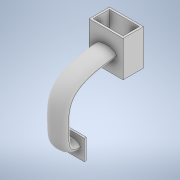
# Autodesk Inventor part: Verbindung_Motor_Servo
Saved by Autodesk Inventor 2021 (Build 250183000, 183)
## iProperties
Created: 2021-01-04
Part Number: Verbindung_Motor_Servo
Material: Generisch
Document SubType Name: Modeling
Designer: Ctroi
Density: 1 g/cm^3
Appearance: Vorgabe
Author: Ctroi
Autodesk Inventor part; units mm, degrees
ref_plane "YZ Plane" through (0, 0, 0) normal (1, 0, 0) x (0, 1, 0)
ref_plane "XZ Plane" through (0, 0, 0) normal (0, 1, 0) x (-1, 0, 0)
ref_plane "XY Plane" through (0, 0, 0) normal (0, 0, 1) x (1, 0, 0)
sketch "Skizze1" plane through (0, 0, 0) normal (0, 1, 0) x (-1, 0, 0)
  line L0 (25, -15) -> (-25, -15)
  line L1 (-25, -15) -> (-25, 15)
  line L2 (-25, 15) -> (25, 15)
  line L3 (25, 15) -> (25, -15)
  line L4 (35, 0) -> (-35, 0) projected
  line L5 (0, -21) -> (0, 21) projected
  point P0 (0, 0)
  dimension "d0" = 50
  dimension "d1" = 30
  constraints: 8 end point, 2 parallel, 1 horizontal, 1 perpendicular, 2 other
  measures "d0" distance of L1.end L2.end
  measures "d1" distance of L0.end L1.end
extrude "Extrusion1" add sketch "Skizze1" along normal blind 3
sketch "Skizze2" plane through (0, 3, 0) normal (0, 1, 0) x (1, 0, 0)
  line L0 (25, -15) -> (25, 15) projected
  line L1 (-25, 15) -> (-25, -15) projected
  line L2 (25, 15) -> (-25, 15)
  line L3 (-25, 15) -> (-25, -15)
  line L4 (-25, -15) -> (25, -15)
  line L5 (25, -15) -> (25, 15)
  line L6 (-22, 12) -> (22, 12)
  line L7 (22, 12) -> (22, -12)
  line L8 (22, -12) -> (-22, -12)
  line L9 (-22, -12) -> (-22, 12)
  point P0 (0, 0)
  dimension "d4" = 3
  constraints: 16 end point, 4 parallel, 2 perpendicular, 1 horizontal, 3 other
  measures "d4" distance between parallel lines of L2 L6
extrude "Extrusion2" add sketch "Skizze2" along normal blind 50
ref_plane "Arbeitsebene1" through (-25, 0, 65) normal (0, 0, 1) x (1, 0, 0)
sketch "Skizze3" plane through (-25, 0, 65) normal (0, 0, 1) x (1, 0, 0)
  line L0 (4.25, -50) -> (45.75, -50)
  line L1 (45.75, -50) -> (45.75, -80)
  line L2 (45.75, -80) -> (4.25, -80)
  line L3 (4.25, -80) -> (4.25, -50)
  line L4 (25, 0) -> (25, -85.9898)
  line L5 (50, 0) -> (0, 0) projected
  dimension "d8" = 41.5
  dimension "d9" = 30
  dimension "d16" = 50
  constraints: 10 end point, 2 parallel, 1 horizontal, 1 perpendicular, 1 vertical, 1 other
  measures "d8" distance of L1.end L2.end
  measures "d9" distance of L0.end L1.end
  measures "d16" distance between parallel lines of L5 L0
extrude "Extrusion3" add sketch "Skizze3" along normal blind 3
sketch "Skizze4" plane through (-25, 0, 15) normal (0, 0, 1) x (1, 0, 0)
  ellipse E0 centre (25, 25.728) end of major axis (40, 25.728) minor radius 7
  point P0 (25, 0)
  dimension "d12" = 15
  dimension "d13" = 7
  constraints: 1 centre point, 1 other
sketch "Skizze5" plane through (0, 0, 0) normal (1, 0, 0) x (0, 1, 0)
  line L0 (0, 15) -> (53, 15) projected
  line L1 (-50, 68) -> (-80, 68) projected
  spline S0 degree 4 poles (26.5, 15) (14.8164, 132.7794) (-31.2312, 55.9062) (-64.9262, 107.2822) (-65, 68) knots 0 0 0 0 0 1 1 1 1 1
  line L2 (-64.9316, 104.4151) -> (-65.0684, 31.5849) construction
  arc A0 (-58.9876, 94.2678) -> (-59.0863, 41.7098) centre (-4.113, 67.8856) ccw construction
  point P0 (0, 0)
  point P1 (-24.9239, 86.1454)
  point P2 (-55.7289, 84.409)
  constraints: 4 midpoint, 2 end point, 1 centre point, 1 point on circle, 6 other
sweep "Sweeping1" add profiles "Skizze4" path "Skizze5" path curves S0
